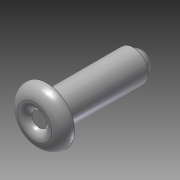
# Autodesk Inventor part: 0.125 Pop Rivet
Saved by Autodesk Inventor 2014 SP1 (Build 180222100, 222)
## iProperties
Created: 2013-12-16
Part Number: 0.125 Pop Rivet
Material: Steel
Document SubType Name: Modeling
Designer: Moses
Density: 7.85 g/cm^3
Appearance: Steel
Mass: 0.736458 g
Surface Area: 2.63469 cm^2
Volume: 0.0938163 cm^3
Author: Moses
Autodesk Inventor part; units mm, degrees
ref_plane "YZ Plane" through (0, 0, 0) normal (1, 0, 0) x (0, 1, 0)
ref_plane "XZ Plane" through (0, 0, 0) normal (0, 1, 0) x (-1, 0, 0)
ref_plane "XY Plane" through (0, 0, 0) normal (0, 0, 1) x (1, 0, 0)
sketch "Sketch1" plane through (0, 0, 0) normal (0, 0, 1) x (1, 0, 0)
  circle A0 centre (0, 0) radius 1.5875
  circle A1 centre (0, 0) radius 2.8575
  circle A2 centre (0, 0) radius 0.889
  dimension "d0" = 3.175
  dimension "d1" = 5.715
  dimension "d2" = 1.778
  constraints: 3 centre point, 3 coincident
  measures "d0" diameter of A0
  measures "d1" diameter of A1
  measures "d2" diameter of A2
extrude "Extrusion1" add sketch "Sketch1" against normal blind 8.89 contours A0
extrude "Extrusion2" add sketch "Sketch1" along normal blind 1.27 contours A0 | A1
fillet "Fillet1" radius 1.27 1 edges at (-2.8575, 0, 1.27)
fillet "Fillet1" radius 0.762 1 edges at (-0.889, 0, 1.27)
sketch "Sketch2" plane through (0, 0, -8.89) normal (0, 0, -1) x (-1, 0, 0)
  circle A0 centre (0, 0) radius 0.889 construction
  circle A1 centre (0, 0) radius 1.5875 projected
  arc A2 (-1.27, 0) -> (1.27, 0) centre (0, 0) ccw
  line L0 (-1.27, 0) -> (1.27, 0)
  circle A3 centre (0, 0) radius 0.762
  dimension "d9" = 2.54
  dimension "d11" = 1.524
  constraints: 4 coincident, 2 centre point, 2 end point, 2 point on circle, 1 horizontal, 1 midpoint
  measures "d9" diameter of A2
  measures "d11" diameter of A3
revolve "Revolution1" add sketch "Sketch2" angle 360 about axis through (1.27, 0, -8.89) along (-1, 0, 0) separate body picked at (-0.1443, -0.209) contours L0 A3 A2 | L0 A3
extrude "Extrusion3" add sketch "Sketch2" against normal blind 9.652 contours A3 L0 | L0 A3 bodies 2
combine bodies "Combine1" operation type subtract main body 1 bodies to subtract 2 keep tools yes
body "Solid1"
body "Solid2"
